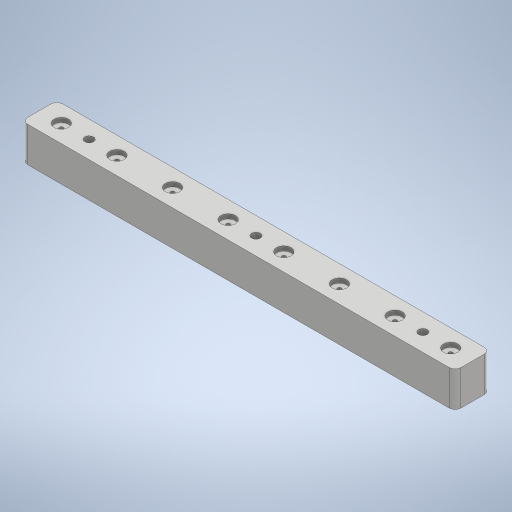
# Autodesk Inventor part: Guia fibra 8Ch V2_2
Saved by Autodesk Inventor 2024 (Build 280153000, 153)
## iProperties
Created: 2024-08-26
Part Number: Guia fibra 8Ch V2_2
Material: Genérico
Document SubType Name: Modeling
Designer: jturizo
Density: 1 g/cm^3
Appearance: Por defecto
Author: jturizo
Autodesk Inventor part; units mm, degrees
ref_plane "YZ Plane" through (0, 0, 0) normal (1, 0, 0) x (0, 1, 0)
ref_plane "XZ Plane" through (0, 0, 0) normal (0, 1, 0) x (-1, 0, 0)
ref_plane "XY Plane" through (0, 0, 0) normal (0, 0, 1) x (1, 0, 0)
sketch "Boceto1" plane through (0, 0, 0) normal (0, 0, 1) x (1, 0, 0)
  line L0 (-74, 6) -> (74, 6)
  line L1 (74, 6) -> (74, -6)
  line L2 (74, -6) -> (-74, -6)
  line L3 (-74, -6) -> (-74, 6)
  circle A0 centre (0, 0) radius 1.5
  circle A1 centre (57, 0) radius 1.5
  circle A2 centre (-57, 0) radius 1.5
  circle A3 centre (-9.5, 0) radius 0.65
  circle A4 centre (9.5, 0) radius 0.65
  circle A5 centre (28.5, 0) radius 0.65
  circle A6 centre (47.5, 0) radius 0.65
  circle A7 centre (66.5, 0) radius 0.65
  circle A8 centre (-28.5, 0) radius 0.65
  circle A9 centre (-47.5, 0) radius 0.65
  circle A10 centre (-66.5, 0) radius 0.65
  point P0 (-74, 0)
  point P1 (0, 6)
  dimension "d0" = 148
  dimension "d1" = 12
  dimension "d2" = 3
  dimension "d3" = 3
  dimension "d4" = 3
  dimension "d5" = 57
  dimension "d6" = 57
  dimension "d7" = 1.3
  dimension "d8" = 1.3
  dimension "d9" = 19
  dimension "d10" = 9.5
  dimension "d13" = 19
  dimension "d20" = 19
  constraints: 11 centre point, 8 end point, 5 horizontal alignment, 3 horizontal, 2 midpoint, 2 parallel, 1 coincident, 1 perpendicular, 1 vertical alignment, 12 other
  measures "d0" distance of L1.end L2.end
  measures "d1" distance of L0.end L1.end
  measures "d2" diameter of A0
  measures "d3" diameter of A1
  measures "d4" diameter of A2
  measures "d5" distance of A1.centre point (0, 0)
  measures "d6" distance of A2.centre point (0, 0)
  measures "d7" diameter of A3
  measures "d8" diameter of A4
  measures "d9" distance of A4.centre A3.centre
  measures "d10" distance of point (0, 0) A3.centre
  measures "d13" distance of A4.centre A5.centre
  measures "d20" distance of A3.centre A8.centre
extrude "Extrusión1" add sketch "Boceto1" along normal blind 12
sketch "Boceto2" plane through (0, 0, 12) normal (0, 0, 1) x (1, 0, 0)
  circle A0 centre (-66.5, 0) radius 0.65 projected
  circle A1 centre (-66.5, 0) radius 2.5
  line L0 (-78, 0) -> (74, 0) construction
  line L1 (74, -6) -> (74, 6) construction
  circle A2 centre (-47.5, 0) radius 2.5
  circle A3 centre (-28.5, 0) radius 2.5
  circle A4 centre (-9.5, 0) radius 2.5
  circle A5 centre (9.5, 0) radius 2.5
  circle A6 centre (28.5, 0) radius 2.5
  circle A7 centre (47.5, 0) radius 2.5
  circle A8 centre (66.5, 0) radius 2.5
  point P0 (0, 0)
  dimension "d27" = 5
  dimension "d30" = 19
  dimension "d35" = 152
  constraints: 8 centre point, 2 end point, 2 horizontal, 1 coincident, 1 midpoint, 14 other
  measures "d27" diameter of A1
  measures "d30" distance of A1.centre A2.centre
  measures "d35" distance from line of L0.start L1
extrude "Extrusión2" cut sketch "Boceto2" against normal blind 1.5 contours A0 | A1 | A2 | A3 | A4 | A5 | A6 | A7 | A8
fillet "Empalme1" radius 2 4 edges at (-74, -6, 6) (74, -6, 6) (74, 6, 6) (-74, 6, 6)
equation "\"d6\" = d5"
equation "\"d8\" = d7"
equation "\"d10\" = 0.5 * d9"
